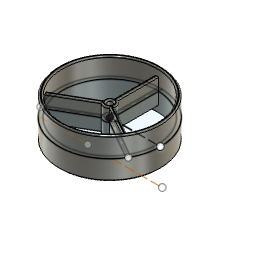
Part_wheel v2 slimmer v2 (Autodesk Fusion 360 design; units mm, degrees)
Autodesk Fusion 360 part; units mm, degrees
note: some values were not read from the file. Set by a fixed rule: which sketch regions a step uses.
sketch "Sketch1" plane through (0, 0, 0) normal (0, 0, 1) x (1, 0, 0)
  circle A0 centre (0, 0) radius 76.2
  circle A1 centre (0, 0) radius 71.2
  circle A2 centre (0, 0) radius 9
  line L0 (0, 0) -> (0, 76.2) construction
  line L1 (0, 0) -> (76.2, 0) construction
  line L2 (0, 0) -> (76.007, 0) construction
  line L3 (2.5, 76.159) -> (2.5, 1.7375)
  line L4 (-2.5, 76.159) -> (-2.5, 0.6433)
  line L5 (55.6203, -52.0848) -> (131.2596, -52.0848) construction
  line L6 (-55.6203, -52.0848) -> (18.9248, -52.0848) construction
  line L7 (0, 0) -> (65.9911, -38.1) construction
  line L8 (0, 0) -> (76.2, 0) construction
  line L9 (0, 0) -> (-65.9911, -38.1) construction
  line L10 (0, 0) -> (76.2, 0) construction
  line L11 (-64.7056, -40.2446) -> (-6.2375, -6.488)
  line L12 (-67.2056, -35.9144) -> (-8.7375, -2.1578)
  line L13 (67.2056, -35.9144) -> (8.7375, -2.1578)
  line L14 (64.7056, -40.2446) -> (6.2375, -6.488)
  circle A3 centre (0, 0) radius 4.175
  dimension "d1" = 152.4
  dimension "d2" = 142.4
  dimension "d3" = 18
  dimension "d10" = 2.5
  dimension "d11" = 2.5
  dimension "d28" = 30
  dimension "d29" = 150
  dimension "d32" = 2.5
  dimension "d33" = 2.5
  dimension "d34" = 2.5
  dimension "d35" = 2.5
  dimension "d40" = 8.35
  constraint coincident A0.centre A1.centre
  constraint concentric A0 A1
  constraint concentric A0 A2
  constraint coincident A0 L0.end
  constraint vertical L0
  constraint horizontal L1
  constraint horizontal L2
  constraint coincident A0 L3.start
  constraint perpendicular L1 L3
  constraint coincident A0 L4.start
  constraint parallel L0 L4
  constraint horizontal L5
  constraint coincident A0 L5.start
  constraint horizontal L6
  constraint coincident A0 L6.start
  constraint horizontal L8
  constraint horizontal L10
  constraint coincident A0 L11.start
  constraint coincident A2 L11.end
  constraint parallel L9 L11
  constraint coincident A0 L12.start
  constraint coincident A2 L12.end
  constraint parallel L9 L12
  constraint coincident A0 L13.start
  constraint coincident A2 L13.end
  constraint parallel L7 L13
  constraint coincident A0 L14.start
  constraint coincident A2 L14.end
  constraint parallel L13 L14
  constraint concentric A0 A3
  measures "d1" diameter of A0
  measures "d2" diameter of A1
  measures "d3" diameter of A2
  measures "d10" distance of L0 L3
  measures "d11" distance of L0 L4
  measures "d28" angle of L7 L8
  measures "d29" angle of L9 L10
  measures "d32" distance of L9 L12
  measures "d33" distance of L9 L11
  measures "d34" distance of L7 L13
  measures "d35" distance of L7 L14
  measures "d40" diameter of A3
extrude "Extrude5" add sketch "Sketch1" along normal blind 30 and the other way blind 30 contours A0 A1 L3 L13 | A0 A1 L3 L4 | A0 A1 L13 L14 | A0 A1 L4 L12 | A0 A1 L11 L14 | A0 A1 L11 L12 makes body 1
extrude "Extrude6" add sketch "Sketch1" along normal blind 20 and the other way blind 20 separate body contours A1 A2 L3 L4 | A1 A2 L13 L14 | A2 L3 L4 A3 | A2 L3 L4 A3 | A1 A2 L11 L12 makes body 2
fillet "Fillet8" radius 2 1 faces at (-6.1572, 74.1049, 30) on bodies 1
fillet "Fillet9" radius 2 1 faces at (-0.2778, 29.4956, 20) on bodies 2
fillet "Fillet10" radius 2 1 faces at (-6.1572, 74.1049, -30) on bodies 1
fillet "Fillet11" radius 2 1 faces at (0.2778, 29.4956, -20) on bodies 2
